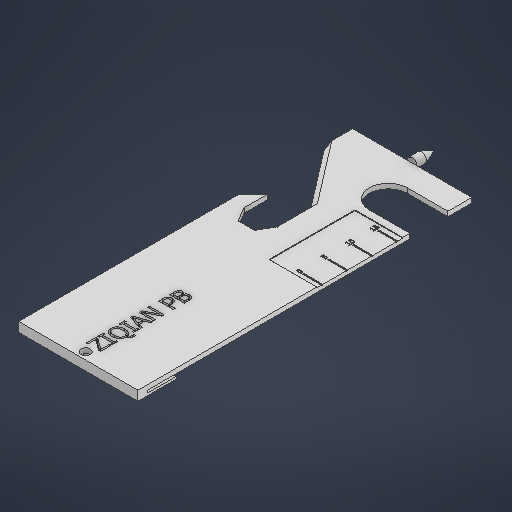
# Autodesk Inventor part: assigment 1
Saved by Autodesk Inventor 2026.1 (Build 301233020, 233B)
## iProperties
Created: 2026-01-31
Part Number: assigment 1
Material: Generic
Document SubType Name: Modeling
Designer: gohzi
Density: 1 g/cm^3
Appearance: Default
Author: gohzi
Autodesk Inventor part; units mm, degrees
ref_plane "YZ Plane" through (0, 0, 0) normal (1, 0, 0) x (0, 1, 0)
ref_plane "XY Plane" through (0, 0, 0) normal (0, 0, 1) x (1, 0, 0)
sketch "Sketch1" plane through (0, 0, 0) normal (0, 1, 0) x (-1, 0, 0)
  line L0 (12.5, 37.5) -> (-12.5, 37.5)
  line L1 (-12.5, 37.5) -> (-12.5, -32.5)
  line L2 (-12.5, -32.5) -> (12.5, -32.5)
  line L3 (12.5, -32.5) -> (12.5, 37.5)
  point P0 (0, 0)
  dimension "d0" = 37.5
  dimension "d1" = 70
  dimension "d2" = 12.5
  dimension "d3" = 12.5
  constraints: 8 end point, 2 parallel, 1 horizontal, 1 perpendicular
  measures "d0" distance from line of point (0, 0) L0
  measures "d1" distance between parallel lines of L2 L0
  measures "d2" distance from line of point (0, 0) L3
  measures "d3" distance from line of L1 point (0, 0)
extrude "Extrusion1" add sketch "Sketch1" along normal blind 1
sketch "Sketch3" plane through (0, 1, 0) normal (0, 1, 0) x (1, 0, 0)
  line L0 (-1.575, -34.5) -> (-1.575, -2.619) construction
  line L1 (-1.575, -2.619) -> (-49.3965, -2.619) construction
  line L2 (-49.3965, -2.619) -> (-49.3965, -34.5) construction
  line L3 (-49.3965, -34.5) -> (-1.575, -34.5) construction
  circle A0 centre (0, -36) radius 1.25 projected
  line L4 (-12.5, -37.5) -> (12.5, -37.5) projected
  line L5 (1.5373, -32.2473) -> (1.5373, -34.3765)
  line L6 (1.5373, -34.3765) -> (1.1593, -34.3765)
  line L7 (1.1593, -34.3765) -> (-1.1501, -32.7463)
  line L8 (-1.1501, -32.7463) -> (-1.1501, -34.3024)
  line L9 (-1.1501, -34.3024) -> (-1.5107, -34.3024)
  line L10 (-1.5107, -34.3024) -> (-1.5107, -32.2893)
  line L11 (-1.5107, -32.2893) -> (-1.1452, -32.2893)
  line L12 (-1.1452, -32.2893) -> (1.1766, -33.9368)
  line L13 (1.1766, -33.9368) -> (1.1766, -32.2473)
  line L14 (1.1766, -32.2473) -> (1.5373, -32.2473)
  line L15 (1.5373, -30.7851) -> (1.5373, -31.9658)
  line L16 (1.5373, -31.9658) -> (1.226, -31.9658)
  line L17 (1.226, -31.9658) -> (1.226, -31.578)
  line L18 (1.226, -31.578) -> (-1.1995, -31.578)
  line L19 (-1.1995, -31.578) -> (-1.1995, -31.9658)
  line L20 (-1.1995, -31.9658) -> (-1.5107, -31.9658)
  line L21 (-1.5107, -31.9658) -> (-1.5107, -30.7851)
  line L22 (-1.5107, -30.7851) -> (-1.1995, -30.7851)
  line L23 (-1.1995, -30.7851) -> (-1.1995, -31.1729)
  line L24 (-1.1995, -31.1729) -> (1.226, -31.1729)
  line L25 (1.226, -31.1729) -> (1.226, -30.7851)
  line L26 (1.226, -30.7851) -> (1.5373, -30.7851)
  spline S0 degree 2 poles (2.2832, -27.7519) (2.3104, -27.8631) (2.34, -28.1051) (2.34, -28.2262) knots 0 0 0 1 2 2 2
  spline S1 degree 2 poles (2.34, -28.2262) (2.34, -28.5695) (1.9572, -28.9968) (1.6015, -29.0166) knots 0 0 0 1 2 2 2
  spline S2 degree 2 poles (1.6015, -29.0166) (1.6015, -29.0437) (1.6015, -29.0907) (1.6015, -29.1104) knots 0 0 0 1 2 2 2
  spline S3 degree 2 poles (1.6015, -29.1104) (1.6015, -29.4192) (1.3915, -29.9156) (1.1865, -30.0935) knots 0 0 0 1 2 2 2
  spline S4 degree 2 poles (1.1865, -30.0935) (0.984, -30.2689) (0.3912, -30.4566) (0.0157, -30.4566) knots 0 0 0 1 2 2 2
  spline S5 degree 2 poles (0.0157, -30.4566) (-0.3696, -30.4566) (-0.9525, -30.2664) (-1.16, -30.091) knots 0 0 0 1 2 2 2
  spline S6 degree 2 poles (-1.16, -30.091) (-1.365, -29.9132) (-1.575, -29.4167) (-1.575, -29.1104) knots 0 0 0 1 2 2 2
  spline S7 degree 2 poles (-1.575, -29.1104) (-1.575, -28.7992) (-1.3576, -28.3003) (-1.16, -28.1274) knots 0 0 0 1 2 2 2
  spline S8 degree 2 poles (-1.16, -28.1274) (-0.9599, -27.9545) (-0.3647, -27.7618) (0.0157, -27.7618) knots 0 0 0 1 2 2 2
  spline S9 degree 2 poles (0.0157, -27.7618) (0.6085, -27.7618) (1.3792, -28.2237) (1.515, -28.6263) knots 0 0 0 1 2 2 2
  spline S10 degree 2 poles (1.515, -28.6263) (1.6287, -28.6164) (1.8114, -28.5571) (1.8633, -28.5102) knots 0 0 0 1 2 2 2
  spline S11 degree 2 poles (1.8633, -28.5102) (1.9275, -28.4534) (1.9868, -28.2978) (1.9868, -28.1595) knots 0 0 0 1 2 2 2
  spline S12 degree 2 poles (1.9868, -28.1595) (1.9868, -28.078) (1.9349, -27.8557) (1.9152, -27.8063) knots 0 0 0 1 2 2 2
  line L27 (1.9152, -27.8063) -> (1.9152, -27.7519)
  line L28 (1.9152, -27.7519) -> (2.2832, -27.7519)
  spline S13 degree 2 poles (0.0157, -28.1842) (-0.2881, -28.1842) (-0.7549, -28.3151) (-0.9081, -28.4336) knots 0 0 0 1 2 2 2
  spline S14 degree 2 poles (-0.9081, -28.4336) (-1.0661, -28.5547) (-1.2242, -28.8955) (-1.2242, -29.108) knots 0 0 0 1 2 2 2
  spline S15 degree 2 poles (-1.2242, -29.108) (-1.2242, -29.3278) (-1.0711, -29.6588) (-0.9081, -29.7847) knots 0 0 0 1 2 2 2
  spline S16 degree 2 poles (-0.9081, -29.7847) (-0.7524, -29.9058) (-0.2807, -30.0342) (0.0157, -30.0342) knots 0 0 0 1 2 2 2
  spline S17 degree 2 poles (0.0157, -30.0342) (0.6159, -30.0342) (1.2557, -29.5303) (1.2557, -29.108) knots 0 0 0 1 2 2 2
  spline S18 degree 2 poles (1.2557, -29.108) (1.2557, -28.6856) (0.6159, -28.1842) (0.0157, -28.1842) knots 0 0 0 1 2 2 2
  line L29 (1.5373, -26.2551) -> (1.5373, -27.4358)
  line L30 (1.5373, -27.4358) -> (1.226, -27.4358)
  line L31 (1.226, -27.4358) -> (1.226, -27.048)
  line L32 (1.226, -27.048) -> (-1.1995, -27.048)
  line L33 (-1.1995, -27.048) -> (-1.1995, -27.4358)
  line L34 (-1.1995, -27.4358) -> (-1.5107, -27.4358)
  line L35 (-1.5107, -27.4358) -> (-1.5107, -26.2551)
  line L36 (-1.5107, -26.2551) -> (-1.1995, -26.2551)
  line L37 (-1.1995, -26.2551) -> (-1.1995, -26.6429)
  line L38 (-1.1995, -26.6429) -> (1.226, -26.6429)
  line L39 (1.226, -26.6429) -> (1.226, -26.2551)
  line L40 (1.226, -26.2551) -> (1.5373, -26.2551)
  line L41 (1.5373, -26.0822) -> (-1.5107, -25.0547)
  line L42 (-1.5107, -25.0547) -> (-1.5107, -24.5557)
  line L43 (-1.5107, -24.5557) -> (1.5373, -23.5282)
  line L44 (1.5373, -23.5282) -> (1.5373, -23.9555)
  line L45 (1.5373, -23.9555) -> (0.6851, -24.2321)
  line L46 (0.6851, -24.2321) -> (0.6851, -25.3955)
  line L47 (0.6851, -25.3955) -> (1.5373, -25.6722)
  line L48 (1.5373, -25.6722) -> (1.5373, -26.0822)
  line L49 (0.3393, -24.3433) -> (-1.0958, -24.8151)
  line L50 (-1.0958, -24.8151) -> (0.3393, -25.2844)
  line L51 (0.3393, -25.2844) -> (0.3393, -24.3433)
  line L52 (1.5373, -21.0582) -> (1.5373, -21.5127)
  line L53 (1.5373, -21.5127) -> (-1.0908, -22.8613)
  line L54 (-1.0908, -22.8613) -> (1.5373, -22.8613)
  line L55 (1.5373, -22.8613) -> (1.5373, -23.2392)
  line L56 (1.5373, -23.2392) -> (-1.5107, -23.2392)
  line L57 (-1.5107, -23.2392) -> (-1.5107, -22.6637)
  line L58 (-1.5107, -22.6637) -> (0.9025, -21.4361)
  line L59 (0.9025, -21.4361) -> (-1.5107, -21.4361)
  line L60 (-1.5107, -21.4361) -> (-1.5107, -21.0582)
  line L61 (-1.5107, -21.0582) -> (1.5373, -21.0582)
  spline S19 degree 2 poles (-0.5919, -17.2049) (-0.3943, -17.2049) (-0.0386, -17.3457) (0.0849, -17.4717) knots 0 0 0 1 2 2 2
  spline S20 degree 2 poles (0.0849, -17.4717) (0.2405, -17.6298) (0.4011, -18.0571) (0.4011, -18.3831) knots 0 0 0 1 2 2 2
  line L62 (0.4011, -18.3831) -> (0.4011, -18.7265)
  line L63 (0.4011, -18.7265) -> (1.5373, -18.7265)
  line L64 (1.5373, -18.7265) -> (1.5373, -19.1316)
  line L65 (1.5373, -19.1316) -> (-1.5107, -19.1316)
  line L66 (-1.5107, -19.1316) -> (-1.5107, -18.3659)
  spline S21 degree 2 poles (-1.5107, -18.3659) (-1.5107, -18.0942) (-1.4218, -17.7138) (-1.3205, -17.568) knots 0 0 0 1 2 2 2
  spline S22 degree 2 poles (-1.3205, -17.568) (-1.2045, -17.3976) (-0.8463, -17.2049) (-0.5919, -17.2049) knots 0 0 0 1 2 2 2
  spline S23 degree 2 poles (-0.5795, -17.6273) (-0.7376, -17.6273) (-0.9698, -17.736) (-1.0439, -17.8472) knots 0 0 0 1 2 2 2
  spline S24 degree 2 poles (-1.0439, -17.8472) (-1.1081, -17.9435) (-1.16, -18.2004) (-1.16, -18.3906) knots 0 0 0 1 2 2 2
  line L67 (-1.16, -18.3906) -> (-1.16, -18.7265)
  line L68 (-1.16, -18.7265) -> (0.0552, -18.7265)
  line L69 (0.0552, -18.7265) -> (0.0552, -18.4498)
  spline S25 degree 2 poles (0.0552, -18.4498) (0.0552, -18.2028) (-0.0238, -17.899) (-0.1275, -17.8002) knots 0 0 0 1 2 2 2
  spline S26 degree 2 poles (-0.1275, -17.8002) (-0.2189, -17.7088) (-0.4338, -17.6273) (-0.5795, -17.6273) knots 0 0 0 1 2 2 2
  spline S27 degree 2 poles (0.6011, -14.7522) (0.8284, -14.7522) (1.1766, -14.9251) (1.2903, -15.0684) knots 0 0 0 1 2 2 2
  spline S28 degree 2 poles (1.2903, -15.0684) (1.4236, -15.2413) (1.5373, -15.634) (1.5373, -15.9452) knots 0 0 0 1 2 2 2
  line L70 (1.5373, -15.9452) -> (1.5373, -16.8196)
  line L71 (1.5373, -16.8196) -> (-1.5107, -16.8196)
  line L72 (-1.5107, -16.8196) -> (-1.5107, -16.0119)
  spline S29 degree 2 poles (-1.5107, -16.0119) (-1.5107, -15.6859) (-1.4688, -15.3598) (-1.3872, -15.2116) knots 0 0 0 1 2 2 2
  spline S30 degree 2 poles (-1.3872, -15.2116) (-1.3008, -15.0462) (-1.0167, -14.8955) (-0.8241, -14.8955) knots 0 0 0 1 2 2 2
  spline S31 degree 2 poles (-0.8241, -14.8955) (-0.6092, -14.8955) (-0.2683, -15.1227) (-0.172, -15.3228) knots 0 0 0 1 2 2 2
  line L73 (-0.172, -15.3228) -> (-0.1572, -15.3228)
  spline S32 degree 2 poles (-0.1572, -15.3228) (-0.0831, -15.0511) (0.3097, -14.7522) (0.6011, -14.7522) knots 0 0 0 1 2 2 2
  spline S33 degree 2 poles (0.6184, -15.1746) (0.4455, -15.1746) (0.2232, -15.2734) (0.1442, -15.4216) knots 0 0 0 1 2 2 2
  spline S34 degree 2 poles (0.1442, -15.4216) (0.0948, -15.5179) (0.0651, -15.7452) (0.0651, -15.9551) knots 0 0 0 1 2 2 2
  line L74 (0.0651, -15.9551) -> (0.0651, -16.4145)
  line L75 (0.0651, -16.4145) -> (1.1915, -16.4145)
  line L76 (1.1915, -16.4145) -> (1.1915, -16.086)
  spline S35 degree 2 poles (1.1915, -16.086) (1.1915, -15.8193) (1.1421, -15.513) (1.063, -15.3944) knots 0 0 0 1 2 2 2
  spline S36 degree 2 poles (1.063, -15.3944) (0.9815, -15.2808) (0.779, -15.1746) (0.6184, -15.1746) knots 0 0 0 1 2 2 2
  spline S37 degree 2 poles (-0.7673, -15.3179) (-0.8759, -15.3179) (-1.039, -15.392) (-1.0859, -15.4735) knots 0 0 0 1 2 2 2
  spline S38 degree 2 poles (-1.0859, -15.4735) (-1.1402, -15.5723) (-1.1649, -15.8119) (-1.1649, -16.0267) knots 0 0 0 1 2 2 2
  line L77 (-1.1649, -16.0267) -> (-1.1649, -16.4145)
  line L78 (-1.1649, -16.4145) -> (-0.2733, -16.4145)
  line L79 (-0.2733, -16.4145) -> (-0.2733, -15.9551)
  spline S39 degree 2 poles (-0.2733, -15.9551) (-0.2733, -15.7649) (-0.3128, -15.5846) (-0.3745, -15.4883) knots 0 0 0 1 2 2 2
  spline S40 degree 2 poles (-0.3745, -15.4883) (-0.4338, -15.3944) (-0.624, -15.3179) (-0.7673, -15.3179) knots 0 0 0 1 2 2 2
  point P0 (0, 0)
  point P1 (0, -37.5)
  dimension "d0" = 37.5
  dimension "d66" = 1.5
  dimension "d74" = 1.5
  constraints: 1 midpoint, 2 other
  measures "d66" distance from line of L3 A0.centre
  measures "d74" distance of A0.centre point (0, -37.5)
ref_plane "Work Plane1" through (0, 1, 0) normal (0, 1, 0) x (-1, 0, 0)
sketch "Sketch13" plane through (0, 1, 0) normal (0, 1, 0) x (-1, 0, 0)
  line L0 (-12.5, -32.5) -> (12.5, -32.5) projected
  line L1 (0, -32.5) -> (-1, -32.5)
  line L2 (-1, -32.5) -> (-1, -34.5)
  line L3 (-1, -34.5) -> (0, -34.5)
  line L4 (0, -34.5) -> (0, -32.5)
  line L5 (-0.1984, -36.5) -> (-1, -34.5)
  line L6 (0, -32.5) -> (0, -36.6739)
  line L7 (0, -36.6739) -> (0, -36.9951)
  line L8 (-0.1984, -36.5) -> (0, -36.9951)
  point P0 (0, 0)
  point P1 (-1, -33.5)
  point P2 (0, -33.5)
  point P3 (-0.5, -32.5)
  point P4 (-0.5, -34.5)
  dimension "d32" = 1
  dimension "d33" = 2
  dimension "d34" = 2
  constraints: 16 end point, 5 midpoint, 2 parallel, 2 point on line, 1 horizontal, 1 perpendicular, 1 vertical
  measures "d32" distance of point (-1, -33.5) point (0, -33.5)
  measures "d33" distance of point (-0.5, -32.5) point (-0.5, -34.5)
  measures "d34" distance from line of L3 L5.start
revolve "Revolution1" add sketch "Sketch13" angle 360 mid plane about axis through (0, 1, -32.5) along (0, 0, -1)
sketch "Sketch15" plane through (0, 1, 0) normal (0, 1, 0) x (1, 0, 0)
  line L0 (0, 32.5) -> (-12.5, 32.5) projected
  line L1 (0, 0) -> (0, 32.5)
  circle A0 centre (4, 23.5) radius 4
  line L2 (12.5, 32.5) -> (0, 32.5) projected
  line L3 (12.5, -37.5) -> (12.5, 32.5) projected
  line L4 (4, 19.5) -> (12.5, 19.5)
  line L5 (12.5, 19.5) -> (12.5, 27.5)
  line L6 (12.5, 27.5) -> (4, 27.5)
  line L7 (4, 27.5) -> (4, 19.5)
  dimension "d47" = 8
  dimension "d48" = 9
  constraints: 10 end point, 2 parallel, 2 vertical, 1 horizontal, 1 perpendicular, 1 point on line, 3 other
  measures "d48" distance from line of L2 point (4, 23.5)
extrude "Extrusion8" cut sketch "Sketch15" against normal blind 10 contours A0 L7 | L6 L3 L4 A0 | A0 L7
sketch "Sketch16" plane through (0, 1, 0) normal (0, 1, 0) x (1, 0, 0)
  line L0 (-12.5, 32.5) -> (-12.5, -37.5) projected
  line L1 (-12.5, 26.5) -> (-2.5718, 13.5618)
  line L2 (-2.5718, 13.5618) -> (-2.5718, 6.7481)
  line L3 (-9.5, 6.7481) -> (-7.7679, 9.7481)
  line L4 (-7.7679, 9.7481) -> (-4.3038, 9.7481)
  line L5 (-4.3038, 9.7481) -> (-2.5718, 6.7481)
  line L6 (-2.5718, 6.7481) -> (-4.3038, 3.7481)
  line L7 (-4.3038, 3.7481) -> (-7.7679, 3.7481)
  line L8 (-7.7679, 3.7481) -> (-9.5, 6.7481)
  line L9 (-9.5, 6.7481) -> (-9.5, 11.7481)
  line L10 (-9.5, 11.7481) -> (-12.5, 11.7481)
  line L11 (-12.5, 26.5) -> (-12.5, 11.7481)
  line L12 (-1, 32.5) -> (-12.5, 32.5) projected
  point P0 (0, 0)
  point P1 (-6.0359, 6.7481)
  point P2 (-6.0359, 9.7481)
  point P3 (-6.0359, 3.7481)
  point P4 (0, 32.5)
  dimension "d55" = 3
  dimension "d56" = 6
  dimension "d65" = 3
  dimension "d67" = 5
  constraints: 22 end point, 2 midpoint, 2 point on line, 1 collinear, 1 parallel, 1 perpendicular, 1 vertical, 13 other
  measures "d55" distance of L9.end L10.end
  measures "d56" distance from line of L12 L1.start
  measures "d65" distance of point (-6.036, 6.748) point (-6.036, 3.748)
  measures "d67" distance of L9.end L3.start
extrude "Extrusion9" cut sketch "Sketch16" against normal blind 2.5
chamfer "Chamfer3" distance 3 angle 45 1 edges at (-12.5, 0.5, -11.7481)
chamfer "Chamfer4" distance 1 angle 45 1 edges at (-7.5359, 1, -20.0309)
sketch "Sketch22" plane through (0, 0, 0) normal (0, -1, 0) x (1, 0, 0)
  line L0 (-12.5, 37.5) -> (12.5, 37.5) projected
  line L1 (12.5, 37.5) -> (12.5, -19.5) projected
  line L2 (-12.5, 37.5) -> (12.5, 37.5)
  line L3 (12.5, 37.5) -> (12.5, 35.5)
  line L4 (12.5, 35.5) -> (-12.5, 35.5)
  line L5 (-12.5, 35.5) -> (-12.5, 37.5)
  point P0 (0, 0)
  dimension "d83" = 2
  constraints: 8 end point, 2 parallel, 1 horizontal, 1 perpendicular, 1 point on line
  measures "d83" distance between parallel lines of L0 L4
extrude "Extrusion14" add sketch "Sketch22" along normal blind 1
sketch "Sketch23" plane through (12.5, 0, 35.5) normal (0, 0, -1) x (-1, 0, 0)
  line L0 (25, -1) -> (0, -1) projected
  line L1 (25, -1) -> (25, 1) projected
  line L2 (0, -1) -> (25, -1)
  line L3 (25, -1) -> (25, -0.5)
  line L4 (25, -0.5) -> (0, -0.5)
  line L5 (0, -0.5) -> (0, -1)
  point P0 (12.5, 0)
  dimension "d86" = 0.5
  constraints: 8 end point, 2 parallel, 1 horizontal, 1 perpendicular, 1 point on line
  measures "d86" distance between parallel lines of L4 L0
extrude "Extrusion15" add sketch "Sketch23" along normal blind 6
sketch "Sketch24" plane through (0, 1, 0) normal (0, 1, 0) x (1, 0, 0)
  circle A0 centre (0, -36) radius 1
  line L0 (-12.5, -37.5) -> (12.5, -37.5) projected
  point P0 (0, 0)
  point P1 (0, -37.5)
  dimension "d89" = 2
  dimension "d90" = 1.5
  constraints: 1 centre point, 1 midpoint
  measures "d89" diameter of A0
  measures "d90" distance of A0.centre point (0, -37.5)
extrude "Extrusion16" cut sketch "Sketch24" against normal blind 6
extrude "Extrusion17" cut sketch "Sketch3" against normal blind 6 contours L5 L6 L7 L8 L9 L10 L11 L12 L13 L14 | L15 L16 L17 L18 L19 L20 L21 L22 L23 L24 L25 L26 | S0 S1 S2 S3 S4 S5 S6 S7 S8 S9 S10 S11 S12 L27 L28 | L29 L30 L31 L32 L33 L34 L35 L36 L37 L38 L39 L40 | L41 L42 L43 L44 L45 L46 L47 L48 | L52 L53 L54 L55 L56 L57 L58 L59 L60 L61 | S19 S20 L62 L63 L64 L65 L66 S21 S22 | S27 S28 L70 L71 L72 S29 S30 S31 L73 S32
sketch "Sketch25" plane through (0, 1, 0) normal (0, 1, 0) x (1, 0, 0)
  line L0 (12.5, -35.5) -> (12.5, 19.5) projected
  line L1 (5.5, 0) -> (12.5, 0)
  line L2 (12.5, 0) -> (12.5, 18)
  line L3 (12.5, 18) -> (5.5, 18)
  line L4 (5.5, 18) -> (5.5, 0)
  line L5 (8.5432, 1) -> (12.5, 1)
  line L6 (12.5, 1) -> (12.5, 1.25)
  line L7 (12.5, 1.25) -> (8.5432, 1.25)
  line L8 (8.5432, 1.25) -> (8.5432, 1)
  line L9 (8.5432, 17) -> (12.5, 17)
  line L10 (12.5, 17) -> (12.5, 16.75)
  line L11 (12.5, 16.75) -> (8.5432, 16.75)
  line L12 (8.5432, 16.75) -> (8.5432, 17)
  line L13 (8.5432, 6.25) -> (12.5, 6.25)
  line L14 (12.5, 6.25) -> (12.5, 6.5)
  line L15 (12.5, 6.5) -> (8.5432, 6.5)
  line L16 (8.5432, 6.5) -> (8.5432, 6.25)
  line L17 (8.5432, 11.5) -> (12.5, 11.5)
  line L18 (12.5, 11.5) -> (12.5, 11.75)
  line L19 (12.5, 11.75) -> (8.5432, 11.75)
  line L20 (8.5432, 11.75) -> (8.5432, 11.5)
  line L21 (8.5432, 16.75) -> (12.5, 16.75)
  line L22 (12.5, 16.75) -> (12.5, 17)
  line L23 (12.5, 17) -> (8.5432, 17)
  line L24 (8.5432, 17) -> (8.5432, 16.75)
  point P0 (0, 0)
  point P1 (9, 18)
  point P2 (10.5216, 17)
  dimension "d95" = 7
  dimension "d96" = 18
  dimension "d97" = 1
  dimension "d98" = 1
  dimension "d99" = 0.25
  dimension "d100" = 0.25
  dimension "d101" = 5
  dimension "d102" = 0.25
  dimension "d103" = 0.25
  dimension "d105" = 0.25
  dimension "d106" = 5
  dimension "d107" = 1
  dimension "d108" = 5
  constraints: 48 end point, 12 parallel, 8 point on line, 6 horizontal, 6 perpendicular, 2 midpoint
  measures "d95" distance between parallel lines of L0 L4
  measures "d96" distance from line of point (9, 18) L1
  measures "d97" distance between parallel lines of L1 L5
  measures "d98" distance between parallel lines of L3 L9
  measures "d99" distance between parallel lines of L7 L5
  measures "d100" distance from line of point (10.522, 17) L11
  measures "d101" distance between parallel lines of L13 L7
  measures "d102" distance between parallel lines of L15 L13
  measures "d103" distance between parallel lines of L19 L17
  measures "d105" distance between parallel lines of L23 L21
  measures "d106" distance between parallel lines of L17 L15
  measures "d107" distance between parallel lines of L3 L23
  measures "d108" distance between parallel lines of L21 L19
extrude "Extrusion18" cut sketch "Sketch25" against normal blind 0.25 contours L5 L8 L7 L0 | L13 L16 L15 L0 | L0 L11 L12 L9 | L17 L20 L19 L0
sketch "Sketch26" plane through (0, 1, 0) normal (0, 1, 0) x (1, 0, 0)
  line L0 (12.5, -37.5) -> (12.5, 1) projected
  line L1 (12.5, 0) -> (2.5, 0)
  line L2 (2.5, 0) -> (2.5, 18)
  line L3 (2.5, 18) -> (12.5, 18)
  line L4 (12.5, 18) -> (12.5, 0)
  point P0 (0, 0)
  point P1 (7.5, 18)
  point P2 (12.5, 1)
  point P3 (12.5, 17)
  dimension "d111" = 18
  dimension "d114" = 10
  constraints: 8 end point, 2 parallel, 1 horizontal, 1 midpoint, 1 perpendicular, 1 point on line
  measures "d111" distance from line of point (7.5, 18) L1
  measures "d114" distance from line of point (12.5, 17) L2
extrude "Extrusion19" cut sketch "Sketch26" against normal blind 0.15
sketch "Sketch28" plane through (0, 1, 0) normal (0, 1, 0) x (1, 0, 0)
  line L0 (7.1987, 6.0409) -> (7.1987, 9.2407) construction
  line L1 (7.1987, 9.2407) -> (11.5687, 9.2407) construction
  line L2 (11.5687, 9.2407) -> (11.5687, 6.0409) construction
  line L3 (11.5687, 6.0409) -> (7.1987, 6.0409) construction
  line L4 (7.1987, 0.7993) -> (7.1987, 1.5497) construction
  line L5 (7.1987, 1.5497) -> (8.2401, 1.5497) construction
  line L6 (8.2401, 1.5497) -> (8.2401, 0.7993) construction
  line L7 (8.2401, 0.7993) -> (7.1987, 0.7993) construction
  line L8 (7.1989, 10.974) -> (7.1986, 12.4748) construction
  line L9 (7.1986, 12.4748) -> (8.2399, 12.475) construction
  line L10 (8.2399, 12.475) -> (8.2402, 10.9742) construction
  line L11 (8.2402, 10.9742) -> (7.1989, 10.974) construction
  line L12 (7.1987, 16.1144) -> (7.1987, 16.7736) construction
  line L13 (7.1987, 16.7736) -> (8.223, 16.7736) construction
  line L14 (8.223, 16.7736) -> (8.223, 16.1144) construction
  line L15 (8.223, 16.1144) -> (7.1987, 16.1144) construction
  spline S0 degree 2 poles (7.719, 1.4946) (7.988, 1.4946) (8.2401, 1.3382) (8.2401, 1.1753) knots 0 0 0 1 2 2 2
  spline S1 degree 2 poles (8.2401, 1.1753) (8.2401, 1.01) (7.9832, 0.8552) (7.7198, 0.8552) knots 0 0 0 1 2 2 2
  spline S2 degree 2 poles (7.7198, 0.8552) (7.4491, 0.8552) (7.1987, 1.0116) (7.1987, 1.1753) knots 0 0 0 1 2 2 2
  spline S3 degree 2 poles (7.1987, 1.1753) (7.1987, 1.3398) (7.4581, 1.4946) (7.719, 1.4946) knots 0 0 0 1 2 2 2
  spline S4 degree 2 poles (8.0237, 1.3228) (7.9743, 1.3422) (7.8219, 1.3584) (7.719, 1.3584) knots 0 0 0 1 2 2 2
  spline S5 degree 2 poles (7.719, 1.3584) (7.6161, 1.3584) (7.4645, 1.3422) (7.4135, 1.322) knots 0 0 0 1 2 2 2
  spline S6 degree 2 poles (7.4135, 1.322) (7.3624, 1.3017) (7.3098, 1.2312) (7.3098, 1.1753) knots 0 0 0 1 2 2 2
  spline S7 degree 2 poles (7.3098, 1.1753) (7.3098, 1.1194) (7.3624, 1.0473) (7.4151, 1.0262) knots 0 0 0 1 2 2 2
  spline S8 degree 2 poles (7.4151, 1.0262) (7.4662, 1.0059) (7.6217, 0.9913) (7.7198, 0.9913) knots 0 0 0 1 2 2 2
  spline S9 degree 2 poles (7.7198, 0.9913) (7.8251, 0.9913) (7.9662, 1.0043) (8.0213, 1.0254) knots 0 0 0 1 2 2 2
  spline S10 degree 2 poles (8.0213, 1.0254) (8.0731, 1.0448) (8.129, 1.117) (8.129, 1.1753) knots 0 0 0 1 2 2 2
  spline S11 degree 2 poles (8.129, 1.1753) (8.129, 1.2304) (8.0764, 1.3025) (8.0237, 1.3228) knots 0 0 0 1 2 2 2
  spline S12 degree 2 poles (7.8811, 6.7199) (7.9532, 6.7199) (8.0764, 6.6738) (8.1217, 6.6316) knots 0 0 0 1 2 2 2
  spline S13 degree 2 poles (8.1217, 6.6316) (8.1671, 6.5895) (8.2198, 6.4639) (8.2198, 6.3861) knots 0 0 0 1 2 2 2
  spline S14 degree 2 poles (8.2198, 6.3861) (8.2198, 6.3148) (8.1882, 6.1754) (8.1631, 6.1243) knots 0 0 0 1 2 2 2
  line L16 (8.1631, 6.1243) -> (8.0213, 6.1243)
  line L17 (8.0213, 6.1243) -> (8.0213, 6.134)
  spline S15 degree 2 poles (8.0213, 6.134) (8.0326, 6.1494) (8.0618, 6.207) (8.0747, 6.2418) knots 0 0 0 1 2 2 2
  spline S16 degree 2 poles (8.0747, 6.2418) (8.0885, 6.2815) (8.1039, 6.3472) (8.1039, 6.3885) knots 0 0 0 1 2 2 2
  spline S17 degree 2 poles (8.1039, 6.3885) (8.1039, 6.429) (8.0747, 6.5052) (8.0431, 6.5328) knots 0 0 0 1 2 2 2
  spline S18 degree 2 poles (8.0431, 6.5328) (8.0132, 6.5579) (7.9337, 6.5838) (7.8803, 6.5838) knots 0 0 0 1 2 2 2
  spline S19 degree 2 poles (7.8803, 6.5838) (7.8268, 6.5838) (7.7587, 6.5546) (7.736, 6.5271) knots 0 0 0 1 2 2 2
  spline S20 degree 2 poles (7.736, 6.5271) (7.7109, 6.4987) (7.6898, 6.4144) (7.6898, 6.3634) knots 0 0 0 1 2 2 2
  spline S21 degree 2 poles (7.6898, 6.3634) (7.6898, 6.3083) (7.7068, 6.1989) (7.7141, 6.1657) knots 0 0 0 1 2 2 2
  line L18 (7.7141, 6.1657) -> (7.1987, 6.1657)
  line L19 (7.1987, 6.1657) -> (7.1987, 6.7143)
  line L20 (7.1987, 6.7143) -> (7.3162, 6.7143)
  line L21 (7.3162, 6.7143) -> (7.3162, 6.2945)
  line L22 (7.3162, 6.2945) -> (7.5828, 6.2945)
  spline S22 degree 2 poles (7.5828, 6.2945) (7.5796, 6.3188) (7.5772, 6.3658) (7.5772, 6.3853) knots 0 0 0 1 2 2 2
  spline S23 degree 2 poles (7.5772, 6.3853) (7.5772, 6.4622) (7.6023, 6.5684) (7.6396, 6.617) knots 0 0 0 1 2 2 2
  spline S24 degree 2 poles (7.6396, 6.617) (7.6769, 6.6665) (7.7903, 6.7199) (7.8811, 6.7199) knots 0 0 0 1 2 2 2
  line L23 (8.219, 11.6136) -> (8.2191, 11.1257)
  line L24 (8.2191, 11.1257) -> (8.117, 11.1257)
  line L25 (8.117, 11.1257) -> (8.117, 11.3072)
  line L26 (8.117, 11.3072) -> (7.4468, 11.3071)
  line L27 (7.4468, 11.3071) -> (7.4468, 11.1256)
  line L28 (7.4468, 11.1256) -> (7.3552, 11.1256)
  spline S25 degree 2 poles (7.3552, 11.1256) (7.3552, 11.2285) (7.2969, 11.3257) (7.2158, 11.3322) knots 0 0 0 1 2 2 2
  line L29 (7.2158, 11.3322) -> (7.2158, 11.4359)
  line L30 (7.2158, 11.4359) -> (8.1169, 11.4361)
  line L31 (8.1169, 11.4361) -> (8.1169, 11.6136)
  line L32 (8.1169, 11.6136) -> (8.219, 11.6136)
  spline S26 degree 2 poles (7.7189, 12.4198) (7.9879, 12.4199) (8.24, 12.2635) (8.24, 12.1006) knots 0 0 0 1 2 2 2
  spline S27 degree 2 poles (8.24, 12.1006) (8.24, 11.9353) (7.9832, 11.7805) (7.7198, 11.7804) knots 0 0 0 1 2 2 2
  spline S28 degree 2 poles (7.7198, 11.7804) (7.4491, 11.7804) (7.1987, 11.9367) (7.1987, 12.1004) knots 0 0 0 1 2 2 2
  spline S29 degree 2 poles (7.1987, 12.1004) (7.1986, 12.2649) (7.4579, 12.4198) (7.7189, 12.4198) knots 0 0 0 1 2 2 2
  spline S30 degree 2 poles (8.0236, 12.2481) (7.9742, 12.2675) (7.8218, 12.2837) (7.7189, 12.2837) knots 0 0 0 1 2 2 2
  spline S31 degree 2 poles (7.7189, 12.2837) (7.616, 12.2837) (7.4644, 12.2674) (7.4134, 12.2472) knots 0 0 0 1 2 2 2
  spline S32 degree 2 poles (7.4134, 12.2472) (7.3623, 12.2269) (7.3097, 12.1564) (7.3097, 12.1005) knots 0 0 0 1 2 2 2
  spline S33 degree 2 poles (7.3097, 12.1005) (7.3097, 12.0445) (7.3624, 11.9724) (7.4151, 11.9514) knots 0 0 0 1 2 2 2
  spline S34 degree 2 poles (7.4151, 11.9514) (7.4661, 11.9311) (7.6217, 11.9166) (7.7198, 11.9166) knots 0 0 0 1 2 2 2
  spline S35 degree 2 poles (7.7198, 11.9166) (7.8251, 11.9166) (7.9661, 11.9296) (8.0212, 11.9507) knots 0 0 0 1 2 2 2
  spline S36 degree 2 poles (8.0212, 11.9507) (8.0731, 11.9701) (8.129, 12.0423) (8.129, 12.1006) knots 0 0 0 1 2 2 2
  spline S37 degree 2 poles (8.129, 12.1006) (8.129, 12.1557) (8.0763, 12.2278) (8.0236, 12.2481) knots 0 0 0 1 2 2 2
  line L33 (8.202, 16.7538) -> (8.202, 16.2659)
  line L34 (8.202, 16.2659) -> (8.0999, 16.2659)
  line L35 (8.0999, 16.2659) -> (8.0999, 16.4474)
  line L36 (8.0999, 16.4474) -> (7.4297, 16.4474)
  line L37 (7.4297, 16.4474) -> (7.4297, 16.2659)
  line L38 (7.4297, 16.2659) -> (7.3381, 16.2659)
  spline S38 degree 2 poles (7.3381, 16.2659) (7.3381, 16.3688) (7.2798, 16.4661) (7.1987, 16.4726) knots 0 0 0 1 2 2 2
  line L39 (7.1987, 16.4726) -> (7.1987, 16.5763)
  line L40 (7.1987, 16.5763) -> (8.0999, 16.5763)
  line L41 (8.0999, 16.5763) -> (8.0999, 16.7538)
  line L42 (8.0999, 16.7538) -> (8.202, 16.7538)
  spline S39 degree 2 poles (7.8843, 17.5439) (7.9564, 17.5439) (8.0796, 17.4977) (8.125, 17.4555) knots 0 0 0 1 2 2 2
  spline S40 degree 2 poles (8.125, 17.4555) (8.1704, 17.4134) (8.223, 17.2878) (8.223, 17.21) knots 0 0 0 1 2 2 2
  spline S41 degree 2 poles (8.223, 17.21) (8.223, 17.1387) (8.1914, 16.9993) (8.1663, 16.9482) knots 0 0 0 1 2 2 2
  line L43 (8.1663, 16.9482) -> (8.0245, 16.9482)
  line L44 (8.0245, 16.9482) -> (8.0245, 16.958)
  spline S42 degree 2 poles (8.0245, 16.958) (8.0358, 16.9734) (8.065, 17.0309) (8.078, 17.0658) knots 0 0 0 1 2 2 2
  spline S43 degree 2 poles (8.078, 17.0658) (8.0918, 17.1055) (8.1072, 17.1711) (8.1072, 17.2124) knots 0 0 0 1 2 2 2
  spline S44 degree 2 poles (8.1072, 17.2124) (8.1072, 17.2529) (8.078, 17.3291) (8.0464, 17.3567) knots 0 0 0 1 2 2 2
  spline S45 degree 2 poles (8.0464, 17.3567) (8.0164, 17.3818) (7.937, 17.4077) (7.8835, 17.4077) knots 0 0 0 1 2 2 2
  spline S46 degree 2 poles (7.8835, 17.4077) (7.83, 17.4077) (7.7619, 17.3786) (7.7393, 17.351) knots 0 0 0 1 2 2 2
  spline S47 degree 2 poles (7.7393, 17.351) (7.7141, 17.3226) (7.6931, 17.2384) (7.6931, 17.1873) knots 0 0 0 1 2 2 2
  spline S48 degree 2 poles (7.6931, 17.1873) (7.6931, 17.1322) (7.7101, 17.0228) (7.7174, 16.9896) knots 0 0 0 1 2 2 2
  line L45 (7.7174, 16.9896) -> (7.202, 16.9896)
  line L46 (7.202, 16.9896) -> (7.202, 17.5382)
  line L47 (7.202, 17.5382) -> (7.3195, 17.5382)
  line L48 (7.3195, 17.5382) -> (7.3195, 17.1184)
  line L49 (7.3195, 17.1184) -> (7.5861, 17.1184)
  spline S49 degree 2 poles (7.5861, 17.1184) (7.5828, 17.1427) (7.5804, 17.1897) (7.5804, 17.2092) knots 0 0 0 1 2 2 2
  spline S50 degree 2 poles (7.5804, 17.2092) (7.5804, 17.2862) (7.6055, 17.3923) (7.6428, 17.441) knots 0 0 0 1 2 2 2
  spline S51 degree 2 poles (7.6428, 17.441) (7.6801, 17.4904) (7.7935, 17.5439) (7.8843, 17.5439) knots 0 0 0 1 2 2 2
  point P0 (0, 0)
  point P1 (7.1987, 1.1745)
  point P2 (7.1987, 11.7244)
  point P3 (7.1987, 16.444)
  dimension "d0" = 37.5
  dimension "d115" = 0
  dimension "d116" = 0
  dimension "d117" = 0
  constraints: 3 midpoint, 8 other
  measures "d115" distance from line of L0 point (7.199, 1.174)
  measures "d116" horizontal distance of point (7.199, 1.174) point (7.199, 11.724)
  measures "d117" horizontal distance of point (7.199, 11.724) point (7.199, 16.444)
extrude "Extrusion20" cut sketch "Sketch28" against normal blind 0.5
equation "\"d57\" = d6"
equation "\"d109\" = d100"
equation "\"d6\" = 2.5"
body "Solid1"
